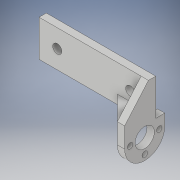
# Autodesk Inventor part: nutHolderX
Saved by Autodesk Inventor 2019 (Build 230136000, 136)
## iProperties
Created: 2019-05-07
Part Number: nutHolderX
Material: Generic
Document SubType Name: Modeling
Designer: Alex Jones
Density: 1 g/cm^3
Appearance: Default
Author: Alex Jones
Autodesk Inventor part; units mm, degrees
ref_plane "YZ Plane" through (0, 0, 0) normal (1, 0, 0) x (0, 1, 0)
sketch "Sketch1" plane through (0, 0, 0) normal (0, 0, 1) x (1, 0, 0)
  circle A0 centre (20, -21.4) radius 2.5 projected
  circle A1 centre (20, 21.4) radius 2.5 projected
  circle A2 centre (-20, -21.4) radius 2.5 projected
  circle A3 centre (-20, 21.4) radius 2.5 projected
  line L0 (-30, 31.4) -> (-30, -31.4) projected
  line L1 (-30, -31.4) -> (30, -31.4) projected
  line L2 (30, -31.4) -> (30, 31.4) projected
  line L3 (30, 31.4) -> (-30, 31.4) projected
  line L4 (-30, -44.5) -> (60, -44.5)
  line L5 (60, -44.5) -> (60, -30.5) projected
  line L6 (-30, -30.5) -> (60, -30.5)
  line L7 (-30, -31.4) -> (30, -31.4)
  line L8 (30, -31.4) -> (30, -11.4)
  line L9 (30, -11.4) -> (-30, -11.4)
  line L10 (-30, -11.4) -> (-30, -31.4)
  line L11 (30, -11.4) -> (-30, -11.4)
  line L12 (-30, -11.4) -> (-30, -28.7084)
  line L13 (-30, -28.7084) -> (30, -28.7084)
  line L14 (30, -28.7084) -> (30, -11.4)
  point P0 (0, 0)
  dimension "d0" = 20
  dimension "d1" = 0
  constraints: 20 end point, 4 horizontal, 4 parallel, 2 perpendicular, 1 point on line, 3 other
  measures "d0" distance between parallel lines of L9 L1
  measures "d1" distance between parallel lines of L2 L8
extrude "Extrusion1" add sketch "Sketch1" along normal blind 4 contours L9 L2 L13 L0
ref_plane "Work Plane1" through (30, -47.6627, 1.8405) normal (-1, 0, 0) x (0, -0.3826834, 0.9238795)
sketch "Sketch2" plane through (30, -47.6627, 1.8405) normal (-1, 0, 0) x (0, -0.3826834, 0.9238795)
  circle A0 centre (0, 11) radius 4 projected
  arc A1 (-10.7913, 13.1327) -> (-9.1051, 17.1723) centre (0, 11) ccw
  line L0 (-5.2583, 18.3379) -> (-11.882, 34.3288) projected
  line L1 (-5.9532, -3.3722) -> (-10.1627, 6.7905)
  line L2 (5.9532, 25.3722) -> (14.3722, 5.0468)
  line L3 (14.3722, 5.0468) -> (-5.9532, -3.3722)
  line L4 (-5.9532, -3.3722) -> (5.9532, 25.3722) construction
  line L5 (-14.3722, 16.9532) -> (14.3722, 5.0468) construction
  line L6 (-7.9238, 14.3204) -> (-13.7905, 11.8904) projected
  line L7 (-7.9238, 14.3204) -> (-31.9564, 72.3401) projected
  line L8 (-4.2095, 21.1627) -> (5.9532, 25.3722)
  line L9 (-28.0775, 29.1357) -> (1.083, -41.2639) projected
  circle A2 centre (7.391, 14.0615) radius 1.5 projected
  circle A3 centre (-7.391, 7.9385) radius 1.5 projected
  circle A4 centre (-3.0615, 18.391) radius 1.5 projected
  circle A5 centre (3.0615, 3.609) radius 1.5 projected
  circle A6 centre (0, 11) radius 4 projected
  circle A7 centre (0, 11) radius 11 projected
  point P0 (-19.9401, 43.3302)
  constraints: 12 end point, 4 point on circle, 3 parallel, 2 midpoint, 2 point on line, 2 tangent, 1 centre point, 1 perpendicular
extrude "Extrusion2" add sketch "Sketch2" along normal blind 4 contours L6 L7 A1 | A1 L3 L1 | A1 L2 L3 | L8 L2 A1
sketch "Sketch3" plane through (30, -11.4, 4) normal (1, 0, 0) x (0, 0, -1)
  line L0 (-13.05, -15.1) -> (-2.05, -15.1) projected
  line L1 (-13.05, -15.1) -> (0, 0)
  arc A0 (0, -15.2927) -> (-2.05, -15.1) centre (-2.05, -26.1) ccw projected
  line L2 (0, 0) -> (0, -15.2927)
  line L3 (0, -15.2927) -> (-13.05, -15.1)
  point P0 (4, 11.4)
  constraints: 6 end point, 1 vertical
extrude "Extrusion3" add sketch "Sketch3" against normal up to surface (4 mm away) contours L1 L2 A0 L0
sketch "Sketch6" plane through (26, -47.6627, 1.8405) normal (-1, 0, 0) x (0, -0.3826834, 0.9238795)
  circle A0 centre (-3.0615, 18.391) radius 1.5 projected
  circle A1 centre (-3.0615, 18.391) radius 2.75
  point P0 (-19.9401, 43.3302)
  dimension "d10" = 5.5
  constraints: 1 centre point, 1 coincident
  measures "d10" diameter of A1
extrude "Extrusion5" add sketch "Sketch6" against normal up to surface (4 mm away) contours A0
sketch "Sketch7" plane through (-30, -28.7084, 0) normal (0, -1, 0) x (1, 0, 0)
  line L0 (56, 17.05) -> (42.95, 4)
  line L1 (0, 4) -> (56, 4) projected
  line L2 (42.95, 4) -> (56, 4)
  line L3 (56, -4.95) -> (56, 17.05) projected
  line L4 (56, 4) -> (56, 17.05)
  point P0 (30, 0)
  dimension "d13" = 45
  constraints: 6 end point, 1 horizontal, 1 perpendicular, 1 point on line
  measures "d13" angle of L1 L0
extrude "Extrusion6" add sketch "Sketch7" against normal up to surface (2.2084 mm away)
sketch "Sketch8" plane through (-30, -28.7084, 0) normal (0, -1, 0) x (1, 0, 0)
  line L0 (56, 0) -> (56, 17.05) projected
  line L1 (56, 17.05) -> (42.95, 4) projected
  line L2 (0, 4) -> (42.95, 4) projected
  line L3 (0, 0) -> (0, 4) projected
  line L4 (0, 0) -> (56, 0) projected
  line L5 (0, 0) -> (56, 0) projected
  line L6 (0, 0) -> (56, 0)
  line L7 (56, 0) -> (56, 4)
  line L8 (56, 4) -> (0, 4)
  line L9 (0, 4) -> (0, 0)
  point P0 (30, 0)
  constraints: 8 end point, 2 parallel, 1 horizontal, 1 perpendicular, 1 point on line
ref_plane "Work Plane2" through (-30, -31.4, -6.35) normal (0, -1, 0) x (1, 0, 0)
extrude "Extrusion7" add sketch "Sketch8" along normal up to surface (2.6916 mm away) contours L4 L3 L2 L8 L0
sketch "Sketch10" plane through (12.95, -28.7084, 4) normal (0, -1, 0) x (1, 0, 0)
  line L0 (0, 0) -> (13.05, 0) projected
  line L1 (13.05, 0) -> (13.05, 13.05) projected
  line L2 (13.05, 13.05) -> (0, 0) projected
  point P0 (-12.95, -4)
extrude "Extrusion8" add sketch "Sketch10" along normal up to surface (2.6916 mm away)
sketch "Sketch12" plane through (26, -47.6627, 1.8405) normal (-1, 0, 0) x (0, -0.3826834, 0.9238795)
  circle A0 centre (7.391, 14.0615) radius 1.5 projected
  circle A1 centre (-7.391, 7.9385) radius 1.5 projected
  circle A2 centre (3.0615, 3.609) radius 1.5 projected
  circle A3 centre (0, 11) radius 4 projected
  line L0 (7.8283, 20.8452) -> (-7.9238, 14.3204) projected
  line L1 (-7.9238, 14.3204) -> (-10.7913, 13.1327) projected
  arc A4 (-10.7913, 13.1327) -> (-10.1627, 6.7905) centre (0, 11) ccw projected
  line L2 (-10.1627, 6.7905) -> (-5.9532, -3.3722) projected
  line L3 (-5.9532, -3.3722) -> (14.3722, 5.0468) projected
  line L4 (14.3722, 5.0468) -> (7.8283, 20.8452) projected
  line L5 (-10.1627, 6.7905) -> (-12.497, 12.4261)
  line L6 (-10.1627, 6.7905) -> (-5.9532, -3.3722) projected
  line L7 (-10.7913, 13.1327) -> (-12.497, 12.4261)
  line L8 (-7.9238, 14.3204) -> (-10.7913, 13.1327) projected
  point P0 (-19.9401, 43.3302)
  constraints: 4 end point, 2 collinear
extrude "Extrusion9" add sketch "Sketch12" against normal up to surface (4 mm away) contours A4 L5 L7
fillet "Fillet1" radius 11 2 edges at (28, -48.5, 17.05) (28, -48.5, -4.95)
sketch "Sketch15" plane through (30, -31.4, 0) normal (1, 0, 0) x (0, 0, -1)
  circle A0 centre (-6.05, -6.1) radius 4 projected
  circle A1 centre (-6.05, -6.1) radius 5.27
  point P0 (0, 31.4)
  dimension "d24" = 1.27
  constraints: 1 centre point
  measures "d24" radial gap between concentric circles of A0 A1
extrude "Extrusion10" cut sketch "Sketch15" against normal through all
body "Solid1"
